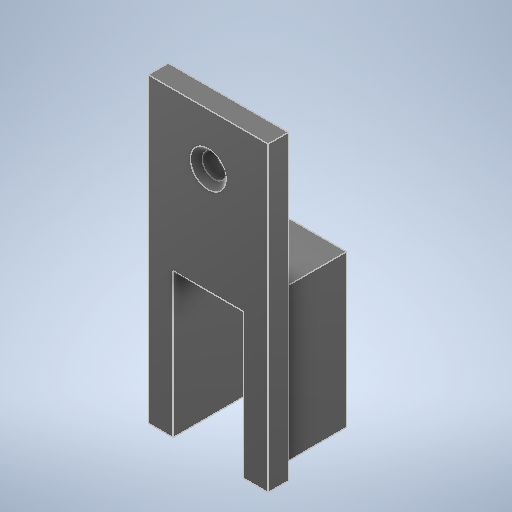
# Autodesk Inventor part: PLU-45 TAPÓN ENCUENTRO CORREDERA (2)
Saved by Autodesk Inventor 2025 (Build 290162000, 162)
## iProperties
Created: 2026-02-23
Part Number: PLU-45 TAPÓN ENCUENTRO CORREDERA (2)
Material: Plástico ABS
Document SubType Name: Modeling
Designer: Frank
Density: 1.06 g/cm^3
Appearance: Suave - Negro
Author: Frank
Autodesk Inventor part; units mm, degrees
ref_plane "YZ Plane" through (0, 0, 0) normal (1, 0, 0) x (0, 1, 0)
ref_plane "XZ Plane" through (0, 0, 0) normal (0, 1, 0) x (-1, 0, 0)
ref_plane "XY Plane" through (0, 0, 0) normal (0, 0, 1) x (1, 0, 0)
sketch "Boceto1" plane through (0, 0, 0) normal (0, 0, 1) x (1, 0, 0)
  line L0 (0, 50.8) -> (-20.2, 50.8)
  line L1 (-20.2, 50.8) -> (-20.2, 0)
  line L2 (-20.2, 0) -> (0, 0)
  line L3 (0, 0) -> (0, 50.8)
  dimension "d0" = 50.8
  dimension "d1" = 20.2
  constraints: 8 end point, 2 parallel, 1 coincident, 1 horizontal, 1 perpendicular
  measures "d0" distance of L0.end L1.end
  measures "d1" distance of L1.end L2.end
extrude "Extrusión1" add sketch "Boceto1" against normal blind 3.4
sketch "Boceto3" plane through (0, 0, 0) normal (0, 0, -1) x (-1, 0, 0)
  line L0 (20.2, 50.8) -> (0, 50.8) construction
  line L1 (0, 50.8) -> (0, 0) construction
  circle A0 centre (10.1, 42.1) radius 2
  line L2 (20.2, 0) -> (20.2, 50.8) projected
  dimension "d20" = 4
  dimension "d21" = 10.1
  dimension "d23" = 8.7
  constraints: 1 centre point
  measures "d20" diameter of A0
  measures "d21" distance from line of L1 A0.centre
  measures "d23" distance from line of L0 A0.centre
hole "Agujero3" at (-10.1, 42.1, 0) direction (0, 0, -1) diameter 4 end through all countersink diameter 6 countersink angle 90
sketch "Boceto6" plane through (0, 0, -3.4) normal (0, 0, -1) x (-1, 0, 0)
  line L0 (0, 0) -> (20.2, 0) projected
  line L1 (2.9, 0) -> (2.9, 25.6)
  line L2 (2.9, 25.6) -> (17.3, 25.6)
  line L3 (17.3, 25.6) -> (17.3, 0)
  line L4 (16, 0) -> (16, 24.3)
  line L5 (16, 24.3) -> (4.2, 24.3)
  line L6 (4.2, 24.3) -> (4.2, 0)
  line L7 (0, 50.8) -> (0, 0) projected
  line L8 (20.2, 0) -> (20.2, 50.8) projected
  circle A0 centre (10.1, 42.1) radius 2 projected
  point P0 (4.2, 0)
  point P1 (16, 0)
  dimension "d40" = 1.3
  dimension "d50" = 14.4
  dimension "d51" = 2.9
  dimension "d52" = 2.9
  dimension "d54" = 25.6
  dimension "d55" = 16.5
  constraints: 12 end point, 4 perpendicular, 2 point on line, 1 vertical, 2 other
  measures "d40" distance between parallel lines of L1 L6
  measures "d50" distance of L1.end L2.end
  measures "d51" distance between parallel lines of L7 L1
  measures "d52" distance between parallel lines of L8 L3
  measures "d54" distance of L1.start L1.end
  measures "d55" distance from line of A0.centre L2
extrude "Extrusión3" add sketch "Boceto6" along normal blind 12.7 contours L1 L2 L3 L0 L4 L5 L6
sketch "Boceto7" plane through (0, 0, -3.4) normal (0, 0, -1) x (-1, 0, 0)
  line L0 (16, 24.3) -> (16, 0) projected
  line L1 (4.2, 24.3) -> (16, 24.3)
  line L2 (16, 24.3) -> (16, 0)
  line L3 (16, 0) -> (4.2, 0)
  line L4 (4.2, 0) -> (4.2, 24.3)
  point P0 (0, 0)
  constraints: 8 end point, 2 parallel, 1 horizontal, 1 perpendicular
extrude "Extrusión4" cut sketch "Boceto7" against normal blind 10
